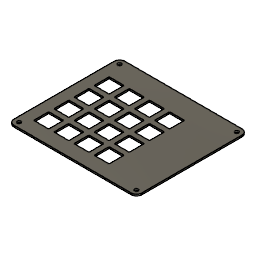
top-plate (Autodesk Fusion 360 design; units mm, degrees)
part number: 2025-12-16-11-07-11-200
Autodesk Fusion 360 part; units mm, degrees
sketch "Sketch1" plane through (0, 0, 0) normal (0, 0, 1) x (1, 0, 0)
  line L0 (-55.6468, 52.0076) -> (65.3532, 52.0076)
  line L1 (65.3532, 52.0076) -> (65.3532, -52.9924)
  line L2 (65.3532, -52.9924) -> (-55.6468, -52.9924)
  line L3 (-55.6468, -52.9924) -> (-55.6468, 52.0076)
  circle A0 centre (-50.6468, 47.0076) radius 1.7
  circle A1 centre (-50.6468, -47.9924) radius 1.7
  circle A2 centre (60.3532, 47.0076) radius 1.7
  circle A3 centre (60.3532, -47.9924) radius 1.7
  line L4 (-44.6468, 31.6576) -> (-31.6468, 31.6576)
  line L5 (-44.6468, 17.6576) -> (-31.6468, 17.6576)
  line L6 (-45.1468, 31.1576) -> (-45.1468, 18.1576)
  line L7 (-31.1468, 31.1576) -> (-31.1468, 18.1576)
  arc A4 (-44.6468, 31.6576) -> (-45.1468, 31.1576) centre (-44.6468, 31.1576) ccw
  arc A5 (-31.1468, 31.1576) -> (-31.6468, 31.6576) centre (-31.6468, 31.1576) ccw
  arc A6 (-45.1468, 18.1576) -> (-44.6468, 17.6576) centre (-44.6468, 18.1576) ccw
  arc A7 (-31.6468, 17.6576) -> (-31.1468, 18.1576) centre (-31.6468, 18.1576) ccw
  line L8 (-25.5968, 31.6576) -> (-12.5968, 31.6576)
  line L9 (-25.5968, 17.6576) -> (-12.5968, 17.6576)
  line L10 (-26.0968, 31.1576) -> (-26.0968, 18.1576)
  line L11 (-12.0968, 31.1576) -> (-12.0968, 18.1576)
  arc A8 (-25.5968, 31.6576) -> (-26.0968, 31.1576) centre (-25.5968, 31.1576) ccw
  arc A9 (-12.0968, 31.1576) -> (-12.5968, 31.6576) centre (-12.5968, 31.1576) ccw
  arc A10 (-26.0968, 18.1576) -> (-25.5968, 17.6576) centre (-25.5968, 18.1576) ccw
  arc A11 (-12.5968, 17.6576) -> (-12.0968, 18.1576) centre (-12.5968, 18.1576) ccw
  line L12 (-6.5468, 31.6576) -> (6.4532, 31.6576)
  line L13 (-6.5468, 17.6576) -> (6.4532, 17.6576)
  line L14 (-7.0468, 31.1576) -> (-7.0468, 18.1576)
  line L15 (6.9532, 31.1576) -> (6.9532, 18.1576)
  arc A12 (-6.5468, 31.6576) -> (-7.0468, 31.1576) centre (-6.5468, 31.1576) ccw
  arc A13 (6.9532, 31.1576) -> (6.4532, 31.6576) centre (6.4532, 31.1576) ccw
  arc A14 (-7.0468, 18.1576) -> (-6.5468, 17.6576) centre (-6.5468, 18.1576) ccw
  arc A15 (6.4532, 17.6576) -> (6.9532, 18.1576) centre (6.4532, 18.1576) ccw
  line L16 (12.5032, 31.6576) -> (25.5032, 31.6576)
  line L17 (12.5032, 17.6576) -> (25.5032, 17.6576)
  line L18 (12.0032, 31.1576) -> (12.0032, 18.1576)
  line L19 (26.0032, 31.1576) -> (26.0032, 18.1576)
  arc A16 (12.5032, 31.6576) -> (12.0032, 31.1576) centre (12.5032, 31.1576) ccw
  arc A17 (26.0032, 31.1576) -> (25.5032, 31.6576) centre (25.5032, 31.1576) ccw
  arc A18 (12.0032, 18.1576) -> (12.5032, 17.6576) centre (12.5032, 18.1576) ccw
  arc A19 (25.5032, 17.6576) -> (26.0032, 18.1576) centre (25.5032, 18.1576) ccw
  line L20 (-44.6468, 12.6076) -> (-31.6468, 12.6076)
  line L21 (-44.6468, -1.3924) -> (-31.6468, -1.3924)
  line L22 (-45.1468, 12.1076) -> (-45.1468, -0.8924)
  line L23 (-31.1468, 12.1076) -> (-31.1468, -0.8924)
  arc A20 (-44.6468, 12.6076) -> (-45.1468, 12.1076) centre (-44.6468, 12.1076) ccw
  arc A21 (-31.1468, 12.1076) -> (-31.6468, 12.6076) centre (-31.6468, 12.1076) ccw
  arc A22 (-45.1468, -0.8924) -> (-44.6468, -1.3924) centre (-44.6468, -0.8924) ccw
  arc A23 (-31.6468, -1.3924) -> (-31.1468, -0.8924) centre (-31.6468, -0.8924) ccw
  line L24 (-25.5968, 12.6076) -> (-12.5968, 12.6076)
  line L25 (-25.5968, -1.3924) -> (-12.5968, -1.3924)
  line L26 (-26.0968, 12.1076) -> (-26.0968, -0.8924)
  line L27 (-12.0968, 12.1076) -> (-12.0968, -0.8924)
  arc A24 (-25.5968, 12.6076) -> (-26.0968, 12.1076) centre (-25.5968, 12.1076) ccw
  arc A25 (-12.0968, 12.1076) -> (-12.5968, 12.6076) centre (-12.5968, 12.1076) ccw
  arc A26 (-26.0968, -0.8924) -> (-25.5968, -1.3924) centre (-25.5968, -0.8924) ccw
  arc A27 (-12.5968, -1.3924) -> (-12.0968, -0.8924) centre (-12.5968, -0.8924) ccw
  line L28 (-6.5468, 12.6076) -> (6.4532, 12.6076)
  line L29 (-6.5468, -1.3924) -> (6.4532, -1.3924)
  line L30 (-7.0468, 12.1076) -> (-7.0468, -0.8924)
  line L31 (6.9532, 12.1076) -> (6.9532, -0.8924)
  arc A28 (-6.5468, 12.6076) -> (-7.0468, 12.1076) centre (-6.5468, 12.1076) ccw
  arc A29 (6.9532, 12.1076) -> (6.4532, 12.6076) centre (6.4532, 12.1076) ccw
  arc A30 (-7.0468, -0.8924) -> (-6.5468, -1.3924) centre (-6.5468, -0.8924) ccw
  arc A31 (6.4532, -1.3924) -> (6.9532, -0.8924) centre (6.4532, -0.8924) ccw
  line L32 (12.5032, 12.6076) -> (25.5032, 12.6076)
  line L33 (12.5032, -1.3924) -> (25.5032, -1.3924)
  line L34 (12.0032, 12.1076) -> (12.0032, -0.8924)
  line L35 (26.0032, 12.1076) -> (26.0032, -0.8924)
  arc A32 (12.5032, 12.6076) -> (12.0032, 12.1076) centre (12.5032, 12.1076) ccw
  arc A33 (26.0032, 12.1076) -> (25.5032, 12.6076) centre (25.5032, 12.1076) ccw
  arc A34 (12.0032, -0.8924) -> (12.5032, -1.3924) centre (12.5032, -0.8924) ccw
  arc A35 (25.5032, -1.3924) -> (26.0032, -0.8924) centre (25.5032, -0.8924) ccw
  line L36 (-44.6468, -6.4424) -> (-31.6468, -6.4424)
  line L37 (-44.6468, -20.4424) -> (-31.6468, -20.4424)
  line L38 (-45.1468, -6.9424) -> (-45.1468, -19.9424)
  line L39 (-31.1468, -6.9424) -> (-31.1468, -19.9424)
  arc A36 (-44.6468, -6.4424) -> (-45.1468, -6.9424) centre (-44.6468, -6.9424) ccw
  arc A37 (-31.1468, -6.9424) -> (-31.6468, -6.4424) centre (-31.6468, -6.9424) ccw
  arc A38 (-45.1468, -19.9424) -> (-44.6468, -20.4424) centre (-44.6468, -19.9424) ccw
  arc A39 (-31.6468, -20.4424) -> (-31.1468, -19.9424) centre (-31.6468, -19.9424) ccw
  line L40 (-25.5968, -6.4424) -> (-12.5968, -6.4424)
  line L41 (-25.5968, -20.4424) -> (-12.5968, -20.4424)
  line L42 (-26.0968, -6.9424) -> (-26.0968, -19.9424)
  line L43 (-12.0968, -6.9424) -> (-12.0968, -19.9424)
  arc A40 (-25.5968, -6.4424) -> (-26.0968, -6.9424) centre (-25.5968, -6.9424) ccw
  arc A41 (-12.0968, -6.9424) -> (-12.5968, -6.4424) centre (-12.5968, -6.9424) ccw
  arc A42 (-26.0968, -19.9424) -> (-25.5968, -20.4424) centre (-25.5968, -19.9424) ccw
  arc A43 (-12.5968, -20.4424) -> (-12.0968, -19.9424) centre (-12.5968, -19.9424) ccw
  line L44 (-6.5468, -6.4424) -> (6.4532, -6.4424)
  line L45 (-6.5468, -20.4424) -> (6.4532, -20.4424)
  line L46 (-7.0468, -6.9424) -> (-7.0468, -19.9424)
  line L47 (6.9532, -6.9424) -> (6.9532, -19.9424)
  arc A44 (-6.5468, -6.4424) -> (-7.0468, -6.9424) centre (-6.5468, -6.9424) ccw
  arc A45 (6.9532, -6.9424) -> (6.4532, -6.4424) centre (6.4532, -6.9424) ccw
  arc A46 (-7.0468, -19.9424) -> (-6.5468, -20.4424) centre (-6.5468, -19.9424) ccw
  arc A47 (6.4532, -20.4424) -> (6.9532, -19.9424) centre (6.4532, -19.9424) ccw
  line L48 (12.5032, -6.4424) -> (25.5032, -6.4424)
  line L49 (12.5032, -20.4424) -> (25.5032, -20.4424)
  line L50 (12.0032, -6.9424) -> (12.0032, -19.9424)
  line L51 (26.0032, -6.9424) -> (26.0032, -19.9424)
  arc A48 (12.5032, -6.4424) -> (12.0032, -6.9424) centre (12.5032, -6.9424) ccw
  arc A49 (26.0032, -6.9424) -> (25.5032, -6.4424) centre (25.5032, -6.9424) ccw
  arc A50 (12.0032, -19.9424) -> (12.5032, -20.4424) centre (12.5032, -19.9424) ccw
  arc A51 (25.5032, -20.4424) -> (26.0032, -19.9424) centre (25.5032, -19.9424) ccw
  line L52 (-44.6468, -25.4924) -> (-31.6468, -25.4924)
  line L53 (-44.6468, -39.4924) -> (-31.6468, -39.4924)
  line L54 (-45.1468, -25.9924) -> (-45.1468, -38.9924)
  line L55 (-31.1468, -25.9924) -> (-31.1468, -38.9924)
  arc A52 (-44.6468, -25.4924) -> (-45.1468, -25.9924) centre (-44.6468, -25.9924) ccw
  arc A53 (-31.1468, -25.9924) -> (-31.6468, -25.4924) centre (-31.6468, -25.9924) ccw
  arc A54 (-45.1468, -38.9924) -> (-44.6468, -39.4924) centre (-44.6468, -38.9924) ccw
  arc A55 (-31.6468, -39.4924) -> (-31.1468, -38.9924) centre (-31.6468, -38.9924) ccw
  line L56 (-25.5968, -25.4924) -> (-12.5968, -25.4924)
  line L57 (-25.5968, -39.4924) -> (-12.5968, -39.4924)
  line L58 (-26.0968, -25.9924) -> (-26.0968, -38.9924)
  line L59 (-12.0968, -25.9924) -> (-12.0968, -38.9924)
  arc A56 (-25.5968, -25.4924) -> (-26.0968, -25.9924) centre (-25.5968, -25.9924) ccw
  arc A57 (-12.0968, -25.9924) -> (-12.5968, -25.4924) centre (-12.5968, -25.9924) ccw
  arc A58 (-26.0968, -38.9924) -> (-25.5968, -39.4924) centre (-25.5968, -38.9924) ccw
  arc A59 (-12.5968, -39.4924) -> (-12.0968, -38.9924) centre (-12.5968, -38.9924) ccw
  line L60 (-6.5468, -25.4924) -> (6.4532, -25.4924)
  line L61 (-6.5468, -39.4924) -> (6.4532, -39.4924)
  line L62 (-7.0468, -25.9924) -> (-7.0468, -38.9924)
  line L63 (6.9532, -25.9924) -> (6.9532, -38.9924)
  arc A60 (-6.5468, -25.4924) -> (-7.0468, -25.9924) centre (-6.5468, -25.9924) ccw
  arc A61 (6.9532, -25.9924) -> (6.4532, -25.4924) centre (6.4532, -25.9924) ccw
  arc A62 (-7.0468, -38.9924) -> (-6.5468, -39.4924) centre (-6.5468, -38.9924) ccw
  arc A63 (6.4532, -39.4924) -> (6.9532, -38.9924) centre (6.4532, -38.9924) ccw
  line L64 (12.5032, -25.4924) -> (25.5032, -25.4924)
  line L65 (12.5032, -39.4924) -> (25.5032, -39.4924)
  line L66 (12.0032, -25.9924) -> (12.0032, -38.9924)
  line L67 (26.0032, -25.9924) -> (26.0032, -38.9924)
  arc A64 (12.5032, -25.4924) -> (12.0032, -25.9924) centre (12.5032, -25.9924) ccw
  arc A65 (26.0032, -25.9924) -> (25.5032, -25.4924) centre (25.5032, -25.9924) ccw
  arc A66 (12.0032, -38.9924) -> (12.5032, -39.4924) centre (12.5032, -38.9924) ccw
  arc A67 (25.5032, -39.4924) -> (26.0032, -38.9924) centre (25.5032, -38.9924) ccw
  dimension "d1" = 121
  dimension "d2" = 105
  dimension "d3" = 3.4
  dimension "d4" = 5
  dimension "d5" = 5
  dimension "d6" = 3.4
  dimension "d7" = 5
  dimension "d8" = 5
  dimension "d9" = 3.4
  dimension "d10" = 5
  dimension "d11" = 5
  dimension "d12" = 3.4
  dimension "d13" = 5
  dimension "d14" = 5
  dimension "d15" = 13.5
  dimension "d16" = 10.5
  dimension "d17" = 13.5
  dimension "d18" = 39.35
  constraint horizontal L0
  constraint vertical L1
  constraint horizontal L2
  constraint vertical L3
  measures "d1" distance of L0.start L0.end
  measures "d2" distance of L0.start L2.end
  measures "d3" diameter of A0
  measures "d4" distance of L0 A0.centre
  measures "d5" distance of L3 A0.centre
  measures "d6" diameter of A1
  measures "d7" distance of L2 A1.centre
  measures "d8" distance of L3 A1.centre
  measures "d9" diameter of A2
  measures "d10" distance of L1 A2.centre
  measures "d11" distance of L0 A2.centre
  measures "d12" diameter of A3
  measures "d13" distance of L2 A3.centre
  measures "d14" distance of L1 A3.centre
  measures "d15" distance of L2 L53
  measures "d16" distance of L3 L54
  measures "d17" distance of L2 L65
  measures "d18" distance of L1 L51
extrude "Extrude1" add sketch "Sketch1" along normal blind 1.5
fillet "Fillet1" radius 5 4 edges at (65.3532, -52.9924, 0.75) (-55.6468, -52.9924, 0.75) (-55.6468, 52.0076, 0.75) (65.3532, 52.0076, 0.75)
